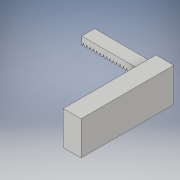
# Autodesk Inventor part: rackPart
Saved by Autodesk Inventor 2019 (Build 230136000, 136)
## iProperties
Created: 2018-11-15
Part Number: rackPart
Material: Generic
Document SubType Name: Modeling
Designer: Charlie
Density: 1 g/cm^3
Appearance: Default
Author: Charlie
Autodesk Inventor part; units mm, degrees
ref_plane "YZ Plane" through (0, 0, 0) normal (1, 0, 0) x (0, 1, 0)
ref_plane "XZ Plane" through (0, 0, 0) normal (0, 1, 0) x (-1, 0, 0)
ref_plane "XY Plane" through (0, 0, 0) normal (0, 0, 1) x (1, 0, 0)
sketch "Sketch1" plane through (0, 0, 0) normal (0, 0, 1) x (1, 0, 0)
  line L0 (0, -5.715) -> (6.35, -5.715)
  line L1 (6.35, -5.715) -> (6.35, 6.35)
  line L2 (6.35, 6.35) -> (0, 6.35)
  line L3 (0, 6.35) -> (0, -5.715)
  point P0 (0, 0)
  dimension "d0" = 6.35
  dimension "d1" = 12.065
  dimension "d2" = 6.35
  dimension "d3" = 6.35
  constraints: 8 end point, 2 parallel, 1 horizontal, 1 perpendicular
  measures "d0" distance of L2.end L1.end
  measures "d1" distance of L1.end L0.end
  measures "d2" distance from line of L2 point (0, 0)
  measures "d3" distance from line of L1 point (0, 0)
extrude "Extrusion1" add sketch "Sketch1" along normal blind 7.62
sketch "Sketch2" plane through (0, -5.715, 0) normal (-1, 0, 0) x (0, 0, 1)
  point P0 (0, 5.715)
sketch "Sketch3" plane through (0, -5.715, 0) normal (-1, 0, 0) x (0, 0, 1)
  line L0 (1.524, 10.795) -> (6.096, 10.795)
  line L1 (6.096, 10.795) -> (6.096, 7.62)
  line L2 (6.096, 7.62) -> (1.524, 7.62)
  line L3 (1.524, 7.62) -> (1.524, 10.795)
  line L4 (0, 12.065) -> (7.62, 12.065) projected
  line L5 (7.62, 12.065) -> (7.62, 0) projected
  line L6 (0, 12.065) -> (0, 0) projected
  point P0 (0, 5.715)
  dimension "d6" = 1.27
  dimension "d7" = 1.524
  dimension "d8" = 1.524
  dimension "d9" = 3.175
  constraints: 8 end point, 2 parallel, 1 horizontal, 1 perpendicular
  measures "d6" distance between parallel lines of L4 L0
  measures "d7" distance between parallel lines of L5 L1
  measures "d8" distance between parallel lines of L6 L3
  measures "d9" distance between parallel lines of L0 L2
extrude "Extrusion2" add sketch "Sketch3" along normal blind 20.32
sketch "Sketch4" plane through (0, 0, 7.62) normal (0, 0, 1) x (1, 0, 0)
  line L0 (6.35, 6.35) -> (0, 6.35) projected
  line L1 (0, 6.35) -> (0, -5.715) projected
  line L2 (0, 6.35) -> (6.35, 6.35)
  line L3 (6.35, 6.35) -> (6.35, -5.715)
  line L4 (6.35, -5.715) -> (0, -5.715)
  line L5 (0, -5.715) -> (0, 6.35)
  point P0 (0, 0)
  point P1 (3.175, 6.35)
  constraints: 8 end point, 2 parallel, 1 horizontal, 1 midpoint, 1 perpendicular
extrude "Extrusion3" add sketch "Sketch4" along normal blind 25.4
sketch "Sketch5" plane through (0, 1.905, 6.096) normal (0, 0, 1) x (1, 0, 0)
  line L0 (0, 0) -> (-20.32, 0) projected
  line L1 (-19.7278, 1.27) -> (-20.32, 0)
  line L2 (-19.7278, 1.27) -> (-19.1356, 0)
  line L3 (-20.32, 0) -> (-19.1356, 0)
  line L4 (-18.5434, 1.27) -> (-19.1356, 0)
  line L5 (-19.1356, 0) -> (-17.9512, 0)
  line L6 (-18.5434, 1.27) -> (-17.9512, 0)
  line L7 (-17.3589, 1.27) -> (-17.9512, 0)
  line L8 (-17.9512, 0) -> (-16.7667, 0)
  line L9 (-17.3589, 1.27) -> (-16.7667, 0)
  line L10 (-16.1745, 1.27) -> (-16.7667, 0)
  line L11 (-16.7667, 0) -> (-15.5823, 0)
  line L12 (-16.1745, 1.27) -> (-15.5823, 0)
  line L13 (-14.9901, 1.27) -> (-15.5823, 0)
  line L14 (-15.5823, 0) -> (-14.3979, 0)
  line L15 (-14.9901, 1.27) -> (-14.3979, 0)
  line L16 (-13.8057, 1.27) -> (-14.3979, 0)
  line L17 (-14.3979, 0) -> (-13.2135, 0)
  line L18 (-13.8057, 1.27) -> (-13.2135, 0)
  line L19 (-12.6213, 1.27) -> (-13.2135, 0)
  line L20 (-13.2135, 0) -> (-12.029, 0)
  line L21 (-12.6213, 1.27) -> (-12.029, 0)
  line L22 (-11.4368, 1.27) -> (-12.029, 0)
  line L23 (-12.029, 0) -> (-10.8446, 0)
  line L24 (-11.4368, 1.27) -> (-10.8446, 0)
  line L25 (-10.2524, 1.27) -> (-10.8446, 0)
  line L26 (-10.8446, 0) -> (-9.6602, 0)
  line L27 (-10.2524, 1.27) -> (-9.6602, 0)
  line L28 (-9.068, 1.27) -> (-9.6602, 0)
  line L29 (-9.6602, 0) -> (-8.4758, 0)
  line L30 (-9.068, 1.27) -> (-8.4758, 0)
  line L31 (-19.7278, 1.27) -> (-19.7278, 0)
  line L32 (-20.32, 0) -> (-20.32, 3.175) projected
  line L33 (-7.8836, 1.27) -> (-8.4758, 0)
  line L34 (-8.4758, 0) -> (-7.2914, 0)
  line L35 (-7.8836, 1.27) -> (-7.2914, 0)
  line L36 (-6.6992, 1.27) -> (-7.2914, 0)
  line L37 (-7.2914, 0) -> (-6.1069, 0)
  line L38 (-6.6992, 1.27) -> (-6.1069, 0)
  line L39 (-5.5147, 1.27) -> (-6.1069, 0)
  line L40 (-6.1069, 0) -> (-4.9225, 0)
  line L41 (-5.5147, 1.27) -> (-4.9225, 0)
  line L42 (-4.3303, 1.27) -> (-4.9225, 0)
  line L43 (-4.9225, 0) -> (-3.7381, 0)
  line L44 (-4.3303, 1.27) -> (-3.7381, 0)
  line L45 (-3.1459, 1.27) -> (-3.7381, 0)
  line L46 (-3.7381, 0) -> (-2.5537, 0)
  line L47 (-3.1459, 1.27) -> (-2.5537, 0)
  line L48 (-1.9615, 1.27) -> (-2.5537, 0)
  line L49 (-2.5537, 0) -> (-1.3693, 0)
  line L50 (-1.9615, 1.27) -> (-1.3693, 0)
  line L51 (-0.777, 1.27) -> (-1.3693, 0)
  line L52 (-1.3693, 0) -> (-0.1848, 0)
  line L53 (-0.777, 1.27) -> (-0.1848, 0)
  point P0 (0, -1.905)
  point P1 (-7.8836, 0)
  point P2 (-6.6992, 0)
  point P3 (-5.5147, 0)
  point P4 (-4.3303, 0)
  point P5 (-3.1459, 0)
  point P6 (-1.9615, 0)
  point P7 (-0.777, 0)
  dimension "d23" = 1.1844
  dimension "d33" = 25
  dimension "d34" = 25
  dimension "d35" = 1.27
  dimension "d36" = 1.1844
  constraints: 104 end point, 1 collinear, 1 horizontal, 1 midpoint, 1 point on line, 102 other
  measures "d23" distance of L1.start L4.start
  measures "d33" angle of L31 L1
  measures "d34" angle of L2 L31
  measures "d35" distance of L31.end L1.start
  measures "d36" distance of L2.end L0.end
extrude "Extrusion6" cut sketch "Sketch5" against normal blind 50.8
sketch "Sketch6" plane through (0, 1.905, 6.096) normal (0, 0, 1) x (1, 0, 0)
  line L0 (-19.7278, 1.27) -> (-19.1356, 0) projected
  line L1 (-18.5434, 1.27) -> (-17.9512, 0) projected
  line L2 (-19.7278, 1.27) -> (-18.5434, 1.27)
  line L3 (-19.1356, 1.27) -> (-19.1356, 0.508)
  circle A0 centre (-19.1356, 0.508) radius 0.2147
  line L4 (-19.1356, 0) -> (-18.5434, 1.27) projected
  line L5 (-19.1356, 0) -> (-18.941, 0.4173)
  line L6 (-19.1356, 0) -> (-19.3302, 0.4173)
  arc A1 (-19.3302, 0.4173) -> (-18.941, 0.4173) centre (-19.1356, 0.508) ccw
  line L7 (-17.9512, 0) -> (-18.1457, 0.4173)
  arc A2 (-18.1457, 0.4173) -> (-17.7566, 0.4173) centre (-17.9512, 0.508) ccw
  line L8 (-17.9512, 0) -> (-17.7566, 0.4173)
  line L9 (-18.5434, 1.27) -> (-17.3589, 1.27)
  line L10 (-16.7667, 0) -> (-16.9613, 0.4173)
  arc A3 (-16.9613, 0.4173) -> (-16.5722, 0.4173) centre (-16.7667, 0.508) ccw
  line L11 (-16.7667, 0) -> (-16.5722, 0.4173)
  line L12 (-17.3589, 1.27) -> (-16.1745, 1.27)
  line L13 (-15.5823, 0) -> (-15.7769, 0.4173)
  arc A4 (-15.7769, 0.4173) -> (-15.3877, 0.4173) centre (-15.5823, 0.508) ccw
  line L14 (-15.5823, 0) -> (-15.3877, 0.4173)
  line L15 (-16.1745, 1.27) -> (-14.9901, 1.27)
  line L16 (-14.3979, 0) -> (-14.5925, 0.4173)
  arc A5 (-14.5925, 0.4173) -> (-14.2033, 0.4173) centre (-14.3979, 0.508) ccw
  line L17 (-14.3979, 0) -> (-14.2033, 0.4173)
  line L18 (-14.9901, 1.27) -> (-13.8057, 1.27)
  line L19 (-13.2135, 0) -> (-13.408, 0.4173)
  arc A6 (-13.408, 0.4173) -> (-13.0189, 0.4173) centre (-13.2135, 0.508) ccw
  line L20 (-13.2135, 0) -> (-13.0189, 0.4173)
  line L21 (-13.8057, 1.27) -> (-12.6213, 1.27)
  line L22 (-12.029, 0) -> (-12.2236, 0.4173)
  arc A7 (-12.2236, 0.4173) -> (-11.8345, 0.4173) centre (-12.029, 0.508) ccw
  line L23 (-12.029, 0) -> (-11.8345, 0.4173)
  line L24 (-12.6213, 1.27) -> (-11.4368, 1.27)
  line L25 (-10.8446, 0) -> (-11.0392, 0.4173)
  arc A8 (-11.0392, 0.4173) -> (-10.6501, 0.4173) centre (-10.8446, 0.508) ccw
  line L26 (-10.8446, 0) -> (-10.6501, 0.4173)
  line L27 (-11.4368, 1.27) -> (-10.2524, 1.27)
  line L28 (-9.6602, 0) -> (-9.8548, 0.4173)
  arc A9 (-9.8548, 0.4173) -> (-9.4656, 0.4173) centre (-9.6602, 0.508) ccw
  line L29 (-9.6602, 0) -> (-9.4656, 0.4173)
  line L30 (-10.2524, 1.27) -> (-9.068, 1.27)
  line L31 (-8.4758, 0) -> (-8.6704, 0.4173)
  arc A10 (-8.6704, 0.4173) -> (-8.2812, 0.4173) centre (-8.4758, 0.508) ccw
  line L32 (-8.4758, 0) -> (-8.2812, 0.4173)
  line L33 (-9.068, 1.27) -> (-7.8836, 1.27)
  line L34 (-7.2914, 0) -> (-7.4859, 0.4173)
  arc A11 (-7.4859, 0.4173) -> (-7.0968, 0.4173) centre (-7.2914, 0.508) ccw
  line L35 (-7.2914, 0) -> (-7.0968, 0.4173)
  line L36 (-7.8836, 1.27) -> (-6.6992, 1.27)
  line L37 (-19.7278, 1.27) -> (-18.5434, 1.27)
  line L38 (-20.32, 0) -> (-20.1254, 0.4173)
  line L39 (-20.32, 0) -> (-20.5146, 0.4173)
  arc A12 (-20.5146, 0.4173) -> (-20.1254, 0.4173) centre (-20.32, 0.508) ccw
  line L40 (-6.1069, 0) -> (-6.3015, 0.4173)
  arc A13 (-6.3015, 0.4173) -> (-5.9124, 0.4173) centre (-6.1069, 0.508) ccw
  line L41 (-6.1069, 0) -> (-5.9124, 0.4173)
  line L42 (-6.6992, 1.27) -> (-5.5147, 1.27)
  line L43 (-4.9225, 0) -> (-5.1171, 0.4173)
  arc A14 (-5.1171, 0.4173) -> (-4.7279, 0.4173) centre (-4.9225, 0.508) ccw
  line L44 (-4.9225, 0) -> (-4.7279, 0.4173)
  line L45 (-5.5147, 1.27) -> (-4.3303, 1.27)
  line L46 (-3.7381, 0) -> (-3.9327, 0.4173)
  arc A15 (-3.9327, 0.4173) -> (-3.5435, 0.4173) centre (-3.7381, 0.508) ccw
  line L47 (-3.7381, 0) -> (-3.5435, 0.4173)
  line L48 (-4.3303, 1.27) -> (-3.1459, 1.27)
  line L49 (-2.5537, 0) -> (-2.7483, 0.4173)
  arc A16 (-2.7483, 0.4173) -> (-2.3591, 0.4173) centre (-2.5537, 0.508) ccw
  line L50 (-2.5537, 0) -> (-2.3591, 0.4173)
  line L51 (-3.1459, 1.27) -> (-1.9615, 1.27)
  line L52 (-1.3693, 0) -> (-1.5638, 0.4173)
  arc A17 (-1.5638, 0.4173) -> (-1.1747, 0.4173) centre (-1.3693, 0.508) ccw
  line L53 (-1.3693, 0) -> (-1.1747, 0.4173)
  line L54 (-1.9615, 1.27) -> (-0.777, 1.27)
  line L55 (-0.1848, 0) -> (-0.3794, 0.4173)
  arc A18 (-0.3794, 0.4173) -> (0.0097, 0.4173) centre (-0.1848, 0.508) ccw
  line L56 (-0.1848, 0) -> (0.0097, 0.4173)
  line L57 (-0.777, 1.27) -> (0.4074, 1.27)
  point P0 (0, -1.905)
  point P1 (-17.9512, 1.27)
  point P2 (-16.7667, 1.27)
  point P3 (-15.5823, 1.27)
  point P4 (-14.3979, 1.27)
  point P5 (-13.2135, 1.27)
  point P6 (-12.029, 1.27)
  point P7 (-10.8446, 1.27)
  point P8 (-9.6602, 1.27)
  point P9 (-8.4758, 1.27)
  point P10 (-7.2914, 1.27)
  point P11 (-6.1069, 1.27)
  point P12 (-4.9225, 1.27)
  point P13 (-3.7381, 1.27)
  point P14 (-2.5537, 1.27)
  point P15 (-1.3693, 1.27)
  point P16 (-0.1848, 1.27)
  dimension "d41" = 0.762
  dimension "d44" = 1.1844
  dimension "d51" = 1.1844
  constraints: 110 end point, 38 point on circle, 19 centre point, 3 horizontal, 2 coincident, 2 point on line, 1 collinear, 1 midpoint, 1 tangent, 1 vertical, 186 other
  measures "d41" distance of L3.start L3.end
  measures "d44" distance of L0.end L7.start
  measures "d51" distance of L9.start L37.start
extrude "Extrusion7" cut sketch "Sketch6" against normal blind 5.08 contours A0 L4 L0 | A2 L8 L1 | L10 A3 L11 | L13 A4 L14 | L16 A5 L17 | L19 A6 L20 | L22 A7 L23 | L25 A8 L26 | L28 A9 L29 | L31 A10 L32 | L34 A11 L35 | L39 A12 L38 | L40 A13 L41 | L43 A14 L44 | L46 A15 L47 | L49 A16 L50 | L52 A17 L53
equation "\"d23\" = d36"
equation "\"d44\" = d36"
equation "\"d51\" = d36"
body "Solid1"
